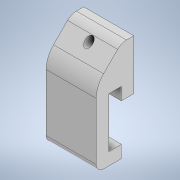
# Autodesk Inventor part: Otwieracz do butelek
Saved by Autodesk Inventor 2021 (Build 250183000, 183)
## iProperties
Created: 2020-04-11
Part Number: Otwieracz do butelek
Material: Ogólny
Document SubType Name: Modeling
Designer: dyrag
Density: 1 g/cm^3
Appearance: Domyślna
Author: dyrag
Autodesk Inventor part; units mm, degrees
ref_plane "YZ Plane" through (0, 0, 0) normal (1, 0, 0) x (0, 1, 0)
ref_plane "XZ Plane" through (0, 0, 0) normal (0, 1, 0) x (-1, 0, 0)
ref_plane "XY Plane" through (0, 0, 0) normal (0, 0, 1) x (1, 0, 0)
sketch "Szkic1" plane through (0, 0, 0) normal (0, 0, 1) x (1, 0, 0)
  line L0 (0, 0) -> (20, 0)
  line L1 (20, 0) -> (20, 20)
  line L2 (20, 20) -> (0, 20)
  line L3 (0, 20) -> (0, 0)
  dimension "d0" = 20
  dimension "d1" = 20
  constraints: 8 end point, 3 perpendicular, 1 horizontal
  measures "d0" distance of L0.start L0.end
  measures "d1" distance of L0.end L1.end
extrude "Wyciągnięcie proste1" add sketch "Szkic1" against normal blind 5
sketch "Szkic2" plane through (0, 0, 0) normal (0, 0, 1) x (1, 0, 0)
  line L0 (0, 0) -> (0, 20) projected
  line L1 (0, 20) -> (0, 5)
  line L2 (0, 5) -> (20, 5)
  line L3 (20, 20) -> (20, 0) projected
  line L4 (20, 5) -> (20, 20)
  line L5 (0, 20) -> (20, 20) projected
  line L6 (20, 20) -> (0, 20)
  dimension "d4" = 15
  constraints: 8 end point, 2 perpendicular, 1 collinear, 1 point on line
  measures "d4" distance of L0.end L1.end
extrude "Wyciągnięcie proste2" add sketch "Szkic2" along normal blind 5
sketch "Szkic3" plane through (0, 0, 5) normal (0, 0, 1) x (1, 0, 0)
  line L0 (0, 20) -> (20, 20) projected
  line L1 (0, 20) -> (0, -25)
  line L2 (0, -25) -> (20, -25)
  line L3 (20, 20) -> (20, 0) projected
  line L4 (20, -25) -> (20, 20)
  line L5 (20, 20) -> (0, 20)
  point P0 (0, 0)
  dimension "d7" = 45
  constraints: 8 end point, 3 perpendicular, 1 vertical
  measures "d7" distance of L0.start L1.end
extrude "Wyciągnięcie proste3" add sketch "Szkic3" along normal blind 5
sketch "Szkic4" plane through (0, 0, 10) normal (0, 0, 1) x (1, 0, 0)
  line L0 (0, -25) -> (0, -20)
  line L1 (0, 5) -> (0, -25) projected
  line L2 (0, -20) -> (20, -20)
  line L3 (20, -25) -> (20, 5) projected
  line L4 (0, -25) -> (20, -25) projected
  line L5 (20, -25) -> (0, -25)
  point P0 (0, 0)
  dimension "d10" = 5
  constraints: 6 end point, 2 point on line, 1 collinear, 1 perpendicular
  measures "d10" distance of L0.start L0.end
extrude "Wyciągnięcie proste4" cut sketch "Szkic4" against normal blind 10
sketch "Szkic5" plane through (0, 0, 5) normal (0, 0, -1) x (-1, 0, 0)
  line L0 (0, 20) -> (0, -20) projected
  line L1 (0, -20) -> (0, -15)
  line L2 (0, -15) -> (-20, -15)
  line L3 (-20, -20) -> (-20, 20) projected
  line L4 (-20, -20) -> (0, -20)
  point P0 (0, 0)
  constraints: 6 end point, 2 perpendicular, 1 point on line
extrude "Wyciągnięcie proste5" add sketch "Szkic5" along normal blind 5
fillet "Zaokrąglenie1" radius 3 1 edges at (10, -20, 10)
chamfer "Faza1" distance 10 angle 45 1 edges at (10, 20, 10)
fillet "Zaokrąglenie2" radius 5 1 edges at (10, 20, 0)
fillet "Zaokrąglenie3" radius 10 1 edges at (10, 10, 10)
sketch "Szkic6" plane through (0, 0, -5) normal (0, 0, -1) x (-1, 0, 0)
  point P0 (0, 0)
  point P1 (-10.1338, 16.9533)
hole "Otwór1" at (10.1338, 16.9533, -5) direction (0, 0, 1) diameter 3 end through all
